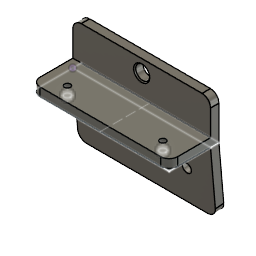
d435_fixed_5deg_mount_v0_1 (Autodesk Fusion 360 design; units mm, degrees)
part number: 2026-05-30-16-41-06-141
Autodesk Fusion 360 part; units mm, degrees
sketch "草图6" plane through (0, 0, 0) normal (0, 1, 0) x (1, 0, 0)
  line L0 (0, 0) -> (65, 0)
  line L1 (65, 0) -> (65, -19.5)
  line L2 (65, -19.5) -> (0, -19.5)
  line L3 (0, -19.5) -> (0, 0)
  line L4 (0, 0) -> (0, 4)
  line L5 (0, 4) -> (65, 4)
  line L6 (65, 4) -> (65, 0)
  circle A0 centre (10, -12.5) radius 1.4
  circle A1 centre (55, -12.5) radius 1.4
  line L7 (32.5, -19.5) -> (32.5, 4) construction
  dimension "d31" = 65
  dimension "d32" = 19.5
  dimension "d33" = 4
  dimension "d34" = 7
  dimension "d35" = 2.8
  dimension "d36" = 45
  constraint horizontal L0
  constraint vertical L1
  constraint horizontal L2
  constraint vertical L3
  constraint coincident L0.start L3.end
  constraint perpendicular L0 L4
  constraint perpendicular L1 L5
  constraint perpendicular L0 L6
  constraint midpoint L2 L7.start
  constraint midpoint L5 L7.end
  constraint symmetric A0 A1 L7
  measures "d31" distance of L0.start L0.end
  measures "d32" distance of L0.start L2.end
  measures "d33" distance of L0.start L4.end
  measures "d34" distance of L2 A0.centre
  measures "d35" diameter of A0
  measures "d36" distance of A0.centre A1.centre
extrude "拉伸5" add sketch "草图6" along normal blind 4 contours L0 L1 L2 L3 makes body 1
extrude "拉伸6" add sketch "草图6" along normal blind 20.105 contours L0 L4 L5 L6 bodies 1
sketch "草图7" plane through (0, 0, 0) normal (0, 0, 1) x (1, 0, 0)
  line L0 (0, 4) -> (65, 4)
  line L1 (65, 4) -> (65, 20.105)
  line L2 (65, 20.105) -> (0, 20.105)
  line L3 (0, 20.105) -> (0, 4)
  circle A0 centre (32.5, 14.15) radius 3.325
  line L4 (32.5, 4) -> (32.5, 20.105) construction
  circle A1 centre (32.5, 14.15) radius 3.825
  dimension "d41" = 10.15
  dimension "d42" = 6.65
  dimension "d43" = 7.65
  constraint midpoint L0 L4.start
  constraint midpoint L2 L4.end
  constraint coincident A0.centre L4
  constraint concentric A0 A1
  measures "d41" distance of L0 A0.centre
  measures "d42" diameter of A0
  measures "d43" diameter of A1
extrude "拉伸7" cut sketch "草图7" against normal blind 4 contours A0 bodies 1
extrude "拉伸8" cut sketch "草图7" against normal blind 0.5 contours A1 bodies 1
chamfer "倒角1" distance 0.5 angle 45 1 edges at (28.9338, 15.5332, -0.5) on bodies 1
fillet "圆角1" radius 4 1 edges at (0, 2, 19.5) on bodies 1
fillet "圆角2" radius 4 1 edges at (65, 2, 19.5) on bodies 1
fillet "圆角3" radius 1 1 edges at (32.5, 4, 0) on bodies 1
fillet "圆角4" radius 4 1 edges at (32.5, 0, -4) on bodies 1
fillet "圆角5" radius 4 1 edges at (0, 20.105, -2) on bodies 1
fillet "圆角6" radius 4 1 edges at (65, 20.105, -2) on bodies 1
delete_face "删除面1" 1 faces at (21.6667, 3.8097, -3.9955) on bodies 1
ref_plane "工作平面1" through (32.5, 0, -4) normal (0, -0.087156, 0.996195) x (1, 0, 0)
sketch "草图8" plane through (0, 0.3473, -3.9696) normal (0, -0.087156, 0.996195) x (1, 0, 0)
  line L0 (0, -0.3486) -> (65, -0.3486)
  line L1 (0, -0.3486) -> (0, -30.3486)
  line L2 (0, -30.3486) -> (65, -30.3486)
  line L3 (65, -30.3486) -> (65, -0.3486)
  line L4 (0, -15.3486) -> (65, -15.3486) construction
  circle A0 centre (12.5, -15.3486) radius 2.15
  line L5 (32.5, -0.3486) -> (32.5, -30.3486) construction
  circle A1 centre (52.5, -15.3486) radius 2.15
  point P0 (0, -0.3486)
  point P1 (65, -0.3486)
  dimension "d62" = 30
  dimension "d64" = 4.3
  dimension "d65" = 40
  constraint horizontal L0
  constraint coincident P0 L0.start
  constraint coincident P1 L0.end
  constraint perpendicular L0 L1
  constraint perpendicular L1 L2
  constraint perpendicular L2 L3
  constraint midpoint L1 L4.start
  constraint midpoint L3 L4.end
  constraint coincident L4 A0.centre
  constraint midpoint L0 L5.start
  constraint midpoint L2 L5.end
  constraint coincident L4 A1.centre
  constraint symmetric A0 L5 A1
  measures "d62" distance of P0 L1.end
  measures "d64" diameter of A0
  measures "d65" distance of A0.centre A1.centre
extrude "拉伸9" add sketch "草图8" along normal blind 4 separate body makes body 2
extrude "拉伸10" add 1 faces at (21.6667, -0.2324, -1.3435) along direction (0, 0.996195, 0.087156) blind 0.877 on bodies 2 bodies 1 2
fillet "圆角7" radius 4 2 edges at (65, -30.0602, -4.6223) (0, -30.0602, -4.6223) on bodies 1
fillet "圆角8" radius 4 1 edges at (32.5, 0, 0.0153) on bodies 1
delete_face "删除面2" 1 faces at (43.3333, -3.2596, -0.2503) on bodies 1
delete_face "删除面3" 1 faces at (21.6667, 4.4199, 0.1854) on bodies 1
extrude "拉伸3" [suppressed]
sketch "草图4" plane through (0, 0, 0) normal (0, 1, 0) x (1, 0, 0)
  line L0 (0, 0) -> (65, 0)
  line L1 (65, 0) -> (65, -25.17)
  line L2 (65, -25.17) -> (0, -25.17)
  line L3 (0, -25.17) -> (0, 0)
  line L4 (0, -7) -> (65, -7) construction
  circle A0 centre (10, -7) radius 1.25
  line L5 (32.5, 0) -> (32.5, -25.17) construction
  circle A1 centre (55, -7) radius 1.25
  line L6 (0, -21.17) -> (65, -21.17)
  dimension "d23" = 25.17
  dimension "d24" = 65
  dimension "d25" = 2.5
  dimension "d26" = 45
  dimension "d27" = 7
  dimension "d28" = 4
  constraint horizontal L0
  constraint vertical L1
  constraint horizontal L2
  constraint vertical L3
  constraint coincident L0.start L3.end
  constraint coincident L4 A0.centre
  constraint midpoint L0 L5.start
  constraint midpoint L2 L5.end
  constraint symmetric A0 L5 A1
  constraint coincident L3 L4.start
  constraint coincident L1 L4.end
  constraint coincident L3 L6.start
  constraint coincident L1 L6.end
  constraint perpendicular L1 L6
  measures "d23" distance of L0.start L2.end
  measures "d24" distance of L0.start L0.end
  measures "d25" diameter of A0
  measures "d26" distance of A0.centre A1.centre
  measures "d27" distance of L0 L4
  measures "d28" distance of L2.end L6.start
extrude "拉伸4" [suppressed]
sketch "草图5" plane through (0, 0, 25.17) normal (0, 0, 1) x (1, 0, 0)
  line L0 (0, 0) -> (65, 0)
  line L1 (65, 0) -> (65, 4)
  line L2 (65, 4) -> (0, 4)
  line L3 (0, 4) -> (0, 0)
equation "d23 = 14 mm + 7.17 mm + 4 mm"
equation "d39 = 16.105 mm + 4 mm"
